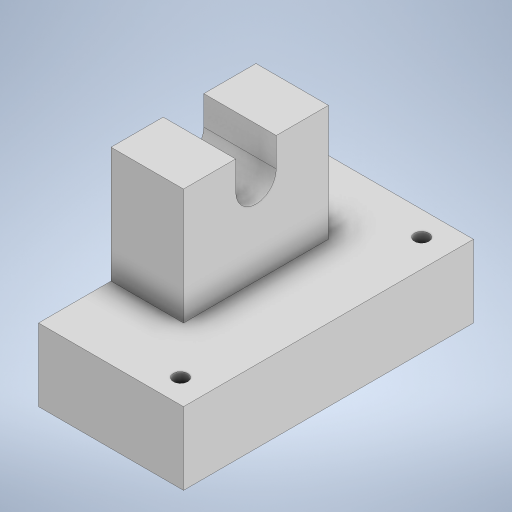
# Autodesk Inventor part: laser_uchwyt
Saved by Autodesk Inventor 2023 (Build 270158000, 158)
## iProperties
Created: 2022-12-18
Part Number: laser_uchwyt
Material: Generic
Document SubType Name: Modeling
Designer: KaczorDonald
Density: 1 g/cm^3
Appearance: Default
Author: KaczorDonald
Autodesk Inventor part; units mm, degrees
ref_plane "YZ Plane" through (0, 0, 0) normal (1, 0, 0) x (0, 1, 0)
ref_plane "XZ Plane" through (0, 0, 0) normal (0, 1, 0) x (-1, 0, 0)
ref_plane "XY Plane" through (0, 0, 0) normal (0, 0, 1) x (1, 0, 0)
sketch "Sketch1" plane through (0, 0, 0) normal (0, 1, 0) x (-1, 0, 0)
  line L0 (0, 0) -> (-10, 0)
  line L1 (-10, 0) -> (-10, 20)
  line L2 (-10, 20) -> (0, 20)
  line L3 (0, 20) -> (0, 0)
  dimension "d0" = 10
  dimension "d1" = 20
  constraints: 8 end point, 2 parallel, 1 horizontal, 1 perpendicular
  measures "d0" distance of L1.end L2.end
  measures "d1" distance of L0.end L1.end
extrude "Extrusion1" add sketch "Sketch1" along normal blind 5
sketch "Sketch2" plane through (0, 5, 0) normal (0, 1, 0) x (1, 0, 0)
  line L0 (0, 0) -> (0, -20) projected
  line L1 (0, -15.0001) -> (5, -15.0001)
  line L2 (5, -15.0001) -> (5, -5.0001)
  line L3 (5, -5.0001) -> (0, -5.0001)
  line L4 (0, -5.0001) -> (0, -15.0001)
  dimension "d4" = 5
  dimension "d5" = 10
  constraints: 8 end point, 2 parallel, 1 horizontal, 1 perpendicular, 1 point on line
  measures "d4" distance of L3.end L2.end
  measures "d5" distance of L2.end L1.end
extrude "Extrusion2" add sketch "Sketch2" along normal blind 8
sketch "Sketch3" plane through (0, 0, 0) normal (-1, 0, 0) x (0, 0, 1)
  circle A0 centre (10.0001, 11.0001) radius 1.5
  point P0 (0, 0)
  dimension "d8" = 3
  constraints: 1 centre point
  measures "d8" diameter of A0
hole "Hole1" at (0, 11.0001, 10.0001) direction (1, 0, 0) diameter 2.8 end through all
sketch "Sketch4" plane through (0, 0, 0) normal (-1, 0, 0) x (0, 0, 1)
  circle A0 centre (10.0001, 11.0001) radius 1.4 projected
  line L0 (15.0001, 13) -> (5.0001, 13) projected
  line L1 (8.6001, 11.0001) -> (11.402, 11.0001)
  line L2 (11.402, 11.0001) -> (11.402, 13)
  line L3 (11.402, 13) -> (8.6001, 13)
  line L4 (8.6001, 13) -> (8.6001, 11.0001)
  point P0 (0, 0)
  constraints: 8 end point, 2 parallel, 1 horizontal, 1 horizontal alignment, 1 perpendicular, 1 point on line, 1 other
extrude "Extrusion3" cut sketch "Sketch4" against normal blind 9.4625 contours L1 A0 | A0 L4 L0 L2 picked at (10.3893, 11.6381)
sketch "Sketch5" plane through (0, 5, 0) normal (0, 1, 0) x (1, 0, 0)
  point P0 (0, 0)
  point P1 (8.0954, -1.6675)
hole "Hole2" at (8.0954, 5, 1.6675) direction (0, -1, 0) diameter 1 end through all
sketch "Sketch6" plane through (0, 5, 0) normal (0, 1, 0) x (1, 0, 0)
  point P0 (0, 0)
  point P1 (8.1579, -18.3637)
hole "Hole3" at (8.1579, 5, 18.3637) direction (0, -1, 0) diameter 1 end through all
body "Solid1"
